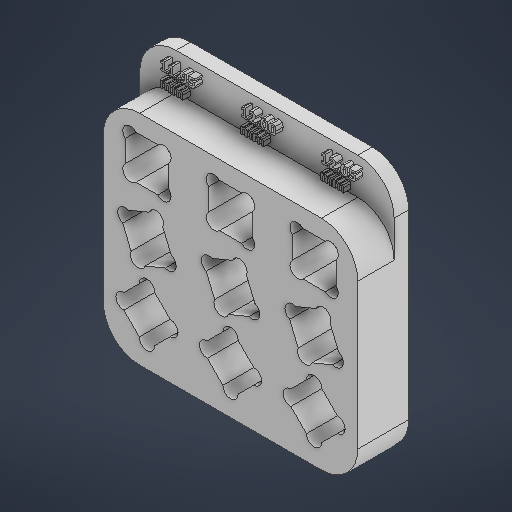
# Autodesk Inventor part: magnet_checker
Saved by Autodesk Inventor 2026.1 (Build 301233020, 233B)
## iProperties
Created: 2025-11-17
Part Number: magnet_checker
Material: Generic
Document SubType Name: Modeling
Designer: Carla Fernandez
Density: 1 g/cm^3
Appearance: Default
Author: Carla Fernandez
Autodesk Inventor part; units mm, degrees
ref_plane "YZ Plane" through (0, 0, 0) normal (1, 0, 0) x (0, 1, 0)
ref_plane "XZ Plane" through (0, 0, 0) normal (0, 1, 0) x (-1, 0, 0)
ref_plane "XY Plane" through (0, 0, 0) normal (0, 0, 1) x (1, 0, 0)
sketch "Sketch1" plane through (0, 0, 0) normal (0, 0, 1) x (1, 0, 0)
  line L0 (-35, 35) -> (35, 35)
  line L1 (35, 35) -> (35, -35)
  line L2 (35, -35) -> (-35, -35)
  line L3 (-35, -35) -> (-35, 35)
  point P0 (0, 0)
  point P1 (0, 35)
  point P2 (35, 0)
  dimension "d0" = 70
  dimension "d1" = 70
  constraints: 8 end point, 2 midpoint, 2 parallel, 1 horizontal, 1 horizontal alignment, 1 perpendicular, 1 vertical alignment
  measures "d0" distance of L2.end L0.start
  measures "d1" distance of L0.start L0.end
extrude "Extrusion1" add sketch "Sketch1" along normal blind 14
sketch "Sketch2" plane through (0, 0, 14) normal (0, 0, 1) x (1, 0, 0)
  line L0 (-28.975, 20) -> (-17.025, 20)
  line L1 (-17.025, 20) -> (-17.025, 8.05)
  line L2 (-17.025, 8.05) -> (-28.975, 8.05)
  line L3 (-28.975, 8.05) -> (-28.975, 20)
  line L4 (-35, 35) -> (-35, -35) projected
  line L5 (35, 35) -> (-35, 35) projected
  line L6 (-30.8067, -0.7414) -> (-19.7664, 3.8317)
  line L7 (-19.7664, 3.8317) -> (-15.1933, -7.2086)
  line L8 (-15.1933, -7.2086) -> (-26.2336, -11.7817)
  line L9 (-26.2336, -11.7817) -> (-30.8067, -0.7414)
  line L10 (-31.4499, -21.975) -> (-23, -13.5251)
  line L11 (-23, -13.5251) -> (-14.5501, -21.975)
  line L12 (-14.5501, -21.975) -> (-23, -30.4249)
  line L13 (-23, -30.4249) -> (-31.4499, -21.975)
  line L14 (-23, -30.4249) -> (-23, -13.5251) construction
  line L15 (-14.5501, -21.975) -> (-31.4499, -21.975) construction
  line L16 (-17.025, 20) -> (-28.975, 8.05) construction
  line L17 (-28.975, 20) -> (-17.025, 8.05) construction
  line L18 (-19.7664, 3.8317) -> (-26.2336, -11.7817) construction
  line L19 (-15.1933, -7.2086) -> (-30.8067, -0.7414) construction
  line L20 (-6, 20.025) -> (6, 20.025)
  line L21 (6, 20.025) -> (6, 8.025)
  line L22 (6, 8.025) -> (-6, 8.025)
  line L23 (-6, 8.025) -> (-6, 20.025)
  line L24 (-7.8394, -0.7278) -> (3.2472, 3.8644)
  line L25 (3.2472, 3.8644) -> (7.8394, -7.2222)
  line L26 (7.8394, -7.2222) -> (-3.2472, -11.8144)
  line L27 (-3.2472, -11.8144) -> (-7.8394, -0.7278)
  line L28 (-8.4853, -21.975) -> (0, -13.4897)
  line L29 (0, -13.4897) -> (8.4853, -21.975)
  line L30 (8.4853, -21.975) -> (0, -30.4603)
  line L31 (0, -30.4603) -> (-8.4853, -21.975)
  line L32 (0, -30.4603) -> (0, -13.4897) construction
  line L33 (8.4853, -21.975) -> (-8.4853, -21.975) construction
  line L34 (6, 20.025) -> (-6, 8.025) construction
  line L35 (-6, 20.025) -> (6, 8.025) construction
  line L36 (3.2472, 3.8644) -> (-3.2472, -11.8144) construction
  line L37 (7.8394, -7.2222) -> (-7.8394, -0.7278) construction
  line L38 (16.975, 20.05) -> (29.025, 20.05)
  line L39 (29.025, 20.05) -> (29.025, 8)
  line L40 (29.025, 8) -> (16.975, 8)
  line L41 (16.975, 8) -> (16.975, 20.05)
  line L42 (15.128, -0.7143) -> (26.2607, 3.897)
  line L43 (26.2607, 3.897) -> (30.872, -7.2357)
  line L44 (30.872, -7.2357) -> (19.7393, -11.847)
  line L45 (19.7393, -11.847) -> (15.128, -0.7143)
  line L46 (14.4794, -21.975) -> (23, -13.4544)
  line L47 (23, -13.4544) -> (31.5206, -21.975)
  line L48 (31.5206, -21.975) -> (23, -30.4956)
  line L49 (23, -30.4956) -> (14.4794, -21.975)
  line L50 (23, -30.4956) -> (23, -13.4544) construction
  line L51 (31.5206, -21.975) -> (14.4794, -21.975) construction
  line L52 (29.025, 20.05) -> (16.975, 8) construction
  line L53 (16.975, 20.05) -> (29.025, 8) construction
  line L54 (26.2607, 3.897) -> (19.7393, -11.847) construction
  line L55 (30.872, -7.2357) -> (15.128, -0.7143) construction
  line L56 (35, -35) -> (35, 35) construction
  point P0 (0, 0)
  point P1 (-23, 14.025)
  point P2 (-23, -21.975)
  point P3 (-23, 14.025)
  point P4 (-23, -3.975)
  point P5 (-23, -21.975)
  point P6 (0, 14.025)
  point P7 (0, -21.975)
  point P8 (0, 14.025)
  point P9 (0, -3.975)
  point P10 (0, -21.975)
  point P11 (23, 14.025)
  point P12 (23, -21.975)
  point P13 (23, 14.025)
  point P14 (23, -3.975)
  point P15 (23, -21.975)
  dimension "d4" = 11.95
  dimension "d6" = 15
  dimension "d9" = 18
  dimension "d10" = 18
  dimension "d11" = 22.5
  dimension "d12" = 12
  dimension "d15" = 18
  dimension "d16" = 18
  dimension "d17" = 22.5
  dimension "d18" = 12.05
  dimension "d21" = 18
  dimension "d22" = 18
  dimension "d23" = 22.5
  dimension "d24" = 12
  dimension "d25" = 12
  constraints: 108 end point, 18 midpoint, 18 parallel, 15 equal length, 15 perpendicular, 7 vertical alignment, 3 horizontal, 3 vertical, 2 horizontal alignment
  measures "d4" distance of L2.end L0.start
  measures "d6" distance between parallel lines of L0 L5
  measures "d9" distance of point (-23, -3.975) point (-23, 14.025)
  measures "d10" distance of point (-23, -21.975) point (-23, -3.975)
  measures "d11" angle of L2 L6
  measures "d12" distance of L23.start L20.start
  measures "d15" distance of point (0, -3.975) point (0, 14.025)
  measures "d16" distance of point (0, -21.975) point (0, -3.975)
  measures "d17" angle of L22 L24
  measures "d18" distance of L41.start L38.start
  measures "d21" distance of point (23, -3.975) point (23, 14.025)
  measures "d22" distance of point (23, -21.975) point (23, -3.975)
  measures "d23" angle of L40 L42
  measures "d24" distance from line of L56 point (23, 14.025)
  measures "d25" distance from line of L4 point (-23, 14.025)
extrude "Extrusion2" cut sketch "Sketch2" against normal blind 12
sketch "Sketch3" plane through (0, 0, 14) normal (0, 0, 1) x (1, 0, 0)
  circle A0 centre (-27.561, 18.586) radius 2.1
  circle A1 centre (-18.439, 18.586) radius 2.1
  circle A2 centre (-27.561, 9.464) radius 2.1
  circle A3 centre (-18.439, 9.464) radius 2.1
  line L0 (-28.975, 20) -> (-17.025, 8.05) construction
  line L1 (-28.975, 8.05) -> (-28.975, 20) construction
  line L2 (-28.975, 20) -> (-17.025, 20) construction
  line L3 (-17.025, 8.05) -> (-28.975, 8.05) construction
  line L4 (-17.025, 20) -> (-28.975, 8.05) construction
  line L5 (-30.8067, -0.7414) -> (-19.7664, 3.8317) construction
  line L6 (-15.1933, -7.2086) -> (-26.2336, -11.7817) construction
  line L7 (-19.7664, 3.8317) -> (-26.2336, -11.7817) construction
  line L8 (-26.2336, -11.7817) -> (-30.8067, -0.7414) construction
  line L9 (-15.1933, -7.2086) -> (-30.8067, -0.7414) construction
  line L10 (-31.4499, -21.975) -> (-23, -13.5251) construction
  line L11 (-23, -30.4249) -> (-31.4499, -21.975) construction
  line L12 (-23, -13.5251) -> (-23, -30.4249) construction
  line L13 (-14.5501, -21.975) -> (-23, -30.4249) construction
  line L14 (-31.4499, -21.975) -> (-14.5501, -21.975) construction
  circle A4 centre (-28.9592, -1.5066) radius 2.1
  circle A5 centre (-20.5316, 1.9842) radius 2.1
  circle A6 centre (-17.0408, -6.4434) radius 2.1
  circle A7 centre (-25.4684, -9.9342) radius 2.1
  line L15 (-19.7664, 3.8317) -> (-15.1933, -7.2086) projected
  circle A8 centre (-23, -15.5248) radius 2.1
  circle A9 centre (-16.5498, -21.975) radius 2.1
  circle A10 centre (-23, -28.4252) radius 2.1
  circle A11 centre (-29.4502, -21.975) radius 2.1
  line L16 (-23, -13.5251) -> (-14.5501, -21.975) projected
  circle A12 centre (-4.561, 18.586) radius 2.1
  circle A13 centre (-4.561, 9.464) radius 2.1
  circle A14 centre (4.561, 9.464) radius 2.1
  line L17 (-5.975, 20) -> (5.975, 8.05) construction
  line L18 (5.975, 20) -> (-5.975, 8.05) construction
  circle A15 centre (4.561, 18.586) radius 2.1
  line L19 (-8.4499, -21.975) -> (8.4499, -21.975) construction
  circle A16 centre (-6.4502, -21.975) radius 2.1
  circle A17 centre (6.4502, -21.975) radius 2.1
  circle A18 centre (0, -28.4252) radius 2.1
  line L20 (0, -13.5251) -> (0, -30.4249) construction
  circle A19 centre (2.4684, 1.9842) radius 2.1
  line L21 (7.8067, -7.2086) -> (-7.8067, -0.7414) construction
  circle A20 centre (5.9592, -6.4434) radius 2.1
  line L22 (3.2336, 3.8317) -> (-3.2336, -11.7817) construction
  circle A21 centre (-2.4684, -9.9342) radius 2.1
  circle A22 centre (0, -15.5248) radius 2.1
  circle A23 centre (-5.9592, -1.5066) radius 2.1
  circle A24 centre (18.439, 18.586) radius 2.1
  circle A25 centre (18.439, 9.464) radius 2.1
  circle A26 centre (27.561, 9.464) radius 2.1
  line L23 (17.025, 20) -> (28.975, 8.05) construction
  line L24 (28.975, 20) -> (17.025, 8.05) construction
  circle A27 centre (27.561, 18.586) radius 2.1
  line L25 (14.5501, -21.975) -> (31.4499, -21.975) construction
  circle A28 centre (16.5498, -21.975) radius 2.1
  circle A29 centre (29.4502, -21.975) radius 2.1
  circle A30 centre (23, -28.4252) radius 2.1
  line L26 (23, -13.5251) -> (23, -30.4249) construction
  circle A31 centre (25.4684, 1.9842) radius 2.1
  line L27 (30.8067, -7.2086) -> (15.1933, -0.7414) construction
  circle A32 centre (28.9592, -6.4434) radius 2.1
  line L28 (26.2336, 3.8317) -> (19.7664, -11.7817) construction
  circle A33 centre (20.5316, -9.9342) radius 2.1
  circle A34 centre (23, -15.5248) radius 2.1
  circle A35 centre (17.0408, -1.5066) radius 2.1
  point P0 (0, 0)
  dimension "d28" = 4.2
  dimension "d29" = 1.414
  dimension "d32" = 1.414
  dimension "d33" = 1.414
  dimension "d34" = 1.414
  dimension "d35" = 1.414
  dimension "d36" = 1.414
  dimension "d37" = 1.414
  dimension "d38" = 1.414
  dimension "d39" = 1.414
  dimension "d42" = 23
  constraints: 36 centre point, 36 end point, 33 point on line, 11 equal radius, 3 coincident, 2 horizontal, 2 horizontal alignment, 2 vertical alignment, 1 vertical, 86 other
  measures "d28" diameter of A0
  measures "d29" distance from line of A0.centre L1
  measures "d32" distance from line of L8 A4.centre
  measures "d33" distance from line of L15 A5.centre
  measures "d34" distance from line of L15 A6.centre
  measures "d35" distance from line of L6 A7.centre
  measures "d36" distance from line of L16 A8.centre
  measures "d37" distance from line of L13 A9.centre
  measures "d38" distance from line of A11.centre L10
  measures "d39" distance from line of L13 A10.centre
  measures "d42" distance of A0.centre A12.centre
extrude "Extrusion3" cut sketch "Sketch3" against normal blind 12
sketch "Sketch4" plane through (0, 0, 14) normal (0, 0, 1) x (1, 0, 0)
  circle A0 centre (-23, 14.025) radius 2
  line L0 (-28.975, 11.0166) -> (-28.975, 17.0334) projected
  line L1 (-26.0084, 20) -> (-19.9916, 20) projected
  circle A1 centre (-23, -3.975) radius 2
  circle A2 centre (-23, -21.975) radius 2
  circle A3 centre (0, 14.025) radius 2
  circle A4 centre (0, -3.975) radius 2
  circle A5 centre (0, -21.975) radius 2
  circle A6 centre (23, 14.025) radius 2
  circle A7 centre (23, -3.975) radius 2
  circle A8 centre (23, -21.975) radius 2
  point P0 (0, 0)
  point P1 (-28.975, 14.025)
  point P2 (-23, 20)
  dimension "d49" = 4
  dimension "d52" = 18
  dimension "d55" = 23
  constraints: 9 centre point, 2 midpoint, 1 horizontal, 1 horizontal alignment, 1 vertical, 1 vertical alignment, 16 other
  measures "d49" diameter of A0
  measures "d52" distance of A0.centre A1.centre
  measures "d55" distance of A0.centre A3.centre
extrude "Extrusion4" cut sketch "Sketch4" against normal through all
sketch "Sketch6" plane through (0, 0, 14) normal (0, 0, 1) x (1, 0, 0)
  line L0 (35, -35) -> (35, 35) projected
  line L1 (-35, 35) -> (35, 35)
  line L2 (35, 35) -> (35, 25)
  line L3 (35, 25) -> (-35, 25)
  line L4 (-35, 25) -> (-35, 35)
  point P0 (0, 0)
  dimension "d60" = 10
  constraints: 8 end point, 2 parallel, 1 horizontal, 1 perpendicular, 1 point on line
  measures "d60" distance between parallel lines of L3 L1
extrude "Extrusion5" cut sketch "Sketch6" against normal blind 10
sketch "Sketch5" plane through (0, 0, 4) normal (0, 0, 1) x (1, 0, 0)
  line L0 (-27.5814, 32.7858) -> (-13.7775, 32.7858) construction
  line L1 (-13.7775, 32.7858) -> (-13.7775, 28.2053) construction
  line L2 (-13.7775, 28.2053) -> (-27.5814, 28.2053) construction
  line L3 (-27.5814, 28.2053) -> (-27.5814, 32.7858) construction
  line L4 (-5.411, 32.7858) -> (5.411, 32.7858) construction
  line L5 (5.411, 32.7858) -> (5.411, 28.2053) construction
  line L6 (5.411, 28.2053) -> (-5.411, 28.2053) construction
  line L7 (-5.411, 28.2053) -> (-5.411, 32.7858) construction
  line L8 (16.6095, 32.7858) -> (30.4134, 32.7858) construction
  line L9 (30.4134, 32.7858) -> (30.4134, 28.2053) construction
  line L10 (30.4134, 28.2053) -> (16.6095, 28.2053) construction
  line L11 (16.6095, 28.2053) -> (16.6095, 32.7858) construction
  line L12 (-25.5704, 30.1943) -> (-27.248, 30.1943)
  line L13 (-27.248, 30.1943) -> (-27.248, 30.6369)
  line L14 (-27.248, 30.6369) -> (-26.7128, 30.6369)
  line L15 (-26.7128, 30.6369) -> (-26.7128, 31.981)
  line L16 (-26.7128, 31.981) -> (-27.248, 31.981)
  line L17 (-27.248, 31.981) -> (-27.248, 32.3947)
  spline S0 degree 2 poles (-27.248, 32.3947) (-27.1306, 32.3947) (-26.898, 32.4256) (-26.8281, 32.4585) knots 0 0 0 1 2 2 2
  spline S1 degree 2 poles (-26.8281, 32.4585) (-26.7478, 32.4997) (-26.6572, 32.6376) (-26.649, 32.7405) knots 0 0 0 1 2 2 2
  line L18 (-26.649, 32.7405) -> (-26.0932, 32.7405)
  line L19 (-26.0932, 32.7405) -> (-26.0932, 30.6369)
  line L20 (-26.0932, 30.6369) -> (-25.5704, 30.6369)
  line L21 (-25.5704, 30.6369) -> (-25.5704, 30.1943)
  line L22 (-23.3453, 30.1943) -> (-25.0229, 30.1943)
  line L23 (-25.0229, 30.1943) -> (-25.0229, 30.6369)
  line L24 (-25.0229, 30.6369) -> (-24.4877, 30.6369)
  line L25 (-24.4877, 30.6369) -> (-24.4877, 31.981)
  line L26 (-24.4877, 31.981) -> (-25.0229, 31.981)
  line L27 (-25.0229, 31.981) -> (-25.0229, 32.3947)
  spline S2 degree 2 poles (-25.0229, 32.3947) (-24.9056, 32.3947) (-24.673, 32.4256) (-24.603, 32.4585) knots 0 0 0 1 2 2 2
  spline S3 degree 2 poles (-24.603, 32.4585) (-24.5227, 32.4997) (-24.4321, 32.6376) (-24.4239, 32.7405) knots 0 0 0 1 2 2 2
  line L28 (-24.4239, 32.7405) -> (-23.8682, 32.7405)
  line L29 (-23.8682, 32.7405) -> (-23.8682, 30.6369)
  line L30 (-23.8682, 30.6369) -> (-23.3453, 30.6369)
  line L31 (-23.3453, 30.6369) -> (-23.3453, 30.1943)
  line L32 (-22.2853, 30.1943) -> (-22.8884, 30.1943)
  line L33 (-22.8884, 30.1943) -> (-22.8884, 30.8653)
  line L34 (-22.8884, 30.8653) -> (-22.2853, 30.8653)
  line L35 (-22.2853, 30.8653) -> (-22.2853, 30.1943)
  spline S4 degree 2 poles (-19.982, 31.6063) (-19.982, 31.2832) (-20.1323, 30.7439) (-20.2908, 30.5504) knots 0 0 0 1 2 2 2
  spline S5 degree 2 poles (-20.2908, 30.5504) (-20.4554, 30.3549) (-20.9412, 30.1449) (-21.2952, 30.1449) knots 0 0 0 1 2 2 2
  spline S6 degree 2 poles (-21.2952, 30.1449) (-21.4146, 30.1449) (-21.674, 30.1758) (-21.7172, 30.1881) knots 0 0 0 1 2 2 2
  line L36 (-21.7172, 30.1881) -> (-21.7172, 30.6863)
  line L37 (-21.7172, 30.6863) -> (-21.6678, 30.6863)
  spline S7 degree 2 poles (-21.6678, 30.6863) (-21.6204, 30.6616) (-21.4434, 30.608) (-21.2891, 30.608) knots 0 0 0 1 2 2 2
  spline S8 degree 2 poles (-21.2891, 30.608) (-21.1635, 30.608) (-20.9309, 30.6739) (-20.8486, 30.746) knots 0 0 0 1 2 2 2
  spline S9 degree 2 poles (-20.8486, 30.746) (-20.7601, 30.8221) (-20.6448, 31.0465) (-20.6242, 31.2153) knots 0 0 0 1 2 2 2
  spline S10 degree 2 poles (-20.6242, 31.2153) (-20.7601, 31.1309) (-20.9947, 31.0403) (-21.1697, 31.0403) knots 0 0 0 1 2 2 2
  spline S11 degree 2 poles (-21.1697, 31.0403) (-21.2993, 31.0403) (-21.5402, 31.1103) (-21.639, 31.1844) knots 0 0 0 1 2 2 2
  spline S12 degree 2 poles (-21.639, 31.1844) (-21.7707, 31.2852) (-21.9251, 31.6084) (-21.9251, 31.8636) knots 0 0 0 1 2 2 2
  spline S13 degree 2 poles (-21.9251, 31.8636) (-21.9251, 32.0633) (-21.7892, 32.3988) (-21.6657, 32.5223) knots 0 0 0 1 2 2 2
  spline S14 degree 2 poles (-21.6657, 32.5223) (-21.5422, 32.6458) (-21.1841, 32.7858) (-20.9638, 32.7858) knots 0 0 0 1 2 2 2
  spline S15 degree 2 poles (-20.9638, 32.7858) (-20.7415, 32.7858) (-20.3978, 32.6623) (-20.2743, 32.5326) knots 0 0 0 1 2 2 2
  spline S16 degree 2 poles (-20.2743, 32.5326) (-20.1302, 32.3885) (-19.982, 31.9316) (-19.982, 31.6063) knots 0 0 0 1 2 2 2
  spline S17 degree 2 poles (-20.6139, 31.701) (-20.6139, 31.9089) (-20.6839, 32.1765) (-20.7477, 32.2506) knots 0 0 0 1 2 2 2
  spline S18 degree 2 poles (-20.7477, 32.2506) (-20.7909, 32.3062) (-20.9021, 32.3535) (-20.9659, 32.3535) knots 0 0 0 1 2 2 2
  spline S19 degree 2 poles (-20.9659, 32.3535) (-21.0235, 32.3535) (-21.1306, 32.3082) (-21.18, 32.2506) knots 0 0 0 1 2 2 2
  spline S20 degree 2 poles (-21.18, 32.2506) (-21.2232, 32.2012) (-21.2849, 32.0098) (-21.2849, 31.8966) knots 0 0 0 1 2 2 2
  spline S21 degree 2 poles (-21.2849, 31.8966) (-21.2849, 31.7731) (-21.2211, 31.6146) (-21.1676, 31.5672) knots 0 0 0 1 2 2 2
  spline S22 degree 2 poles (-21.1676, 31.5672) (-21.112, 31.5199) (-20.9741, 31.4828) (-20.8877, 31.4828) knots 0 0 0 1 2 2 2
  spline S23 degree 2 poles (-20.8877, 31.4828) (-20.8156, 31.4828) (-20.6654, 31.522) (-20.618, 31.5425) knots 0 0 0 1 2 2 2
  spline S24 degree 2 poles (-20.618, 31.5425) (-20.618, 31.5611) (-20.6139, 31.631) (-20.6139, 31.701) knots 0 0 0 1 2 2 2
  spline S25 degree 2 poles (-17.7487, 31.0547) (-17.7487, 30.855) (-17.8845, 30.5175) (-18.0183, 30.396) knots 0 0 0 1 2 2 2
  spline S26 degree 2 poles (-18.0183, 30.396) (-18.1521, 30.2746) (-18.5185, 30.1408) (-18.7861, 30.1408) knots 0 0 0 1 2 2 2
  spline S27 degree 2 poles (-18.7861, 30.1408) (-19.0702, 30.1429) (-19.4777, 30.2355) (-19.6115, 30.2952) knots 0 0 0 1 2 2 2
  line L38 (-19.6115, 30.2952) -> (-19.6115, 30.8489)
  line L39 (-19.6115, 30.8489) -> (-19.5539, 30.8489)
  spline S28 degree 2 poles (-19.5539, 30.8489) (-19.5045, 30.8221) (-19.3851, 30.7521) (-19.2883, 30.7151) knots 0 0 0 1 2 2 2
  spline S29 degree 2 poles (-19.2883, 30.7151) (-19.1978, 30.6801) (-19.0105, 30.6327) (-18.8973, 30.6327) knots 0 0 0 1 2 2 2
  spline S30 degree 2 poles (-18.8973, 30.6327) (-18.7985, 30.6327) (-18.5679, 30.6821) (-18.4979, 30.748) knots 0 0 0 1 2 2 2
  spline S31 degree 2 poles (-18.4979, 30.748) (-18.4465, 30.7995) (-18.3888, 30.925) (-18.3888, 31.03) knots 0 0 0 1 2 2 2
  spline S32 degree 2 poles (-18.3888, 31.03) (-18.3888, 31.1206) (-18.4629, 31.2482) (-18.5226, 31.2873) knots 0 0 0 1 2 2 2
  spline S33 degree 2 poles (-18.5226, 31.2873) (-18.6091, 31.3449) (-18.8561, 31.3779) (-18.9446, 31.3779) knots 0 0 0 1 2 2 2
  spline S34 degree 2 poles (-18.9446, 31.3779) (-19.0846, 31.3779) (-19.3501, 31.3326) (-19.4468, 31.3079) knots 0 0 0 1 2 2 2
  line L40 (-19.4468, 31.3079) -> (-19.5024, 31.3079)
  line L41 (-19.5024, 31.3079) -> (-19.5024, 32.7343)
  line L42 (-19.5024, 32.7343) -> (-17.8187, 32.7343)
  line L43 (-17.8187, 32.7343) -> (-17.8187, 32.2547)
  line L44 (-17.8187, 32.2547) -> (-18.8993, 32.2547)
  line L45 (-18.8993, 32.2547) -> (-18.8993, 31.8328)
  spline S35 degree 2 poles (-18.8993, 31.8328) (-18.8479, 31.8369) (-18.7058, 31.841) (-18.6667, 31.841) knots 0 0 0 1 2 2 2
  spline S36 degree 2 poles (-18.6667, 31.841) (-18.4835, 31.841) (-18.1748, 31.7669) (-18.0533, 31.6907) knots 0 0 0 1 2 2 2
  spline S37 degree 2 poles (-18.0533, 31.6907) (-17.9092, 31.5961) (-17.7487, 31.2811) (-17.7487, 31.0547) knots 0 0 0 1 2 2 2
  line L46 (-25.0661, 26.0123) -> (-25.0661, 26.9694)
  spline S38 degree 2 poles (-25.0661, 26.9694) (-25.0661, 27.1114) (-25.0764, 27.3049) (-25.1011, 27.3667) knots 0 0 0 1 2 2 2
  spline S39 degree 2 poles (-25.1011, 27.3667) (-25.1279, 27.4284) (-25.2349, 27.484) (-25.3316, 27.484) knots 0 0 0 1 2 2 2
  spline S40 degree 2 poles (-25.3316, 27.484) (-25.3996, 27.484) (-25.5313, 27.4243) (-25.6095, 27.3687) knots 0 0 0 1 2 2 2
  line L47 (-25.6095, 27.3687) -> (-25.6095, 26.0123)
  line L48 (-25.6095, 26.0123) -> (-26.2106, 26.0123)
  line L49 (-26.2106, 26.0123) -> (-26.2106, 26.9694)
  spline S41 degree 2 poles (-26.2106, 26.9694) (-26.2106, 27.1094) (-26.2229, 27.3049) (-26.2476, 27.3667) knots 0 0 0 1 2 2 2
  spline S42 degree 2 poles (-26.2476, 27.3667) (-26.2744, 27.4284) (-26.3814, 27.484) (-26.4781, 27.484) knots 0 0 0 1 2 2 2
  spline S43 degree 2 poles (-26.4781, 27.484) (-26.5502, 27.484) (-26.6922, 27.4161) (-26.7581, 27.3687) knots 0 0 0 1 2 2 2
  line L50 (-26.7581, 27.3687) -> (-26.7581, 26.0123)
  line L51 (-26.7581, 26.0123) -> (-27.355, 26.0123)
  line L52 (-27.355, 26.0123) -> (-27.355, 27.9286)
  line L53 (-27.355, 27.9286) -> (-26.7581, 27.9286)
  line L54 (-26.7581, 27.9286) -> (-26.7581, 27.7166)
  spline S44 degree 2 poles (-26.7581, 27.7166) (-26.6119, 27.8401) (-26.3505, 27.9801) (-26.1879, 27.9801) knots 0 0 0 1 2 2 2
  spline S45 degree 2 poles (-26.1879, 27.9801) (-26.013, 27.9801) (-25.7454, 27.8133) (-25.6754, 27.6466) knots 0 0 0 1 2 2 2
  spline S46 degree 2 poles (-25.6754, 27.6466) (-25.5045, 27.8072) (-25.1999, 27.9801) (-25.0435, 27.9801) knots 0 0 0 1 2 2 2
  spline S47 degree 2 poles (-25.0435, 27.9801) (-24.9097, 27.9801) (-24.6977, 27.8957) (-24.6256, 27.8092) knots 0 0 0 1 2 2 2
  spline S48 degree 2 poles (-24.6256, 27.8092) (-24.5454, 27.7166) (-24.4651, 27.4634) (-24.4651, 27.2596) knots 0 0 0 1 2 2 2
  line L55 (-24.4651, 27.2596) -> (-24.4651, 26.0123)
  line L56 (-24.4651, 26.0123) -> (-25.0661, 26.0123)
  line L57 (-21.7357, 26.0123) -> (-21.7357, 26.9694)
  spline S49 degree 2 poles (-21.7357, 26.9694) (-21.7357, 27.1114) (-21.746, 27.3049) (-21.7707, 27.3667) knots 0 0 0 1 2 2 2
  spline S50 degree 2 poles (-21.7707, 27.3667) (-21.7975, 27.4284) (-21.9045, 27.484) (-22.0012, 27.484) knots 0 0 0 1 2 2 2
  spline S51 degree 2 poles (-22.0012, 27.484) (-22.0692, 27.484) (-22.2009, 27.4243) (-22.2791, 27.3687) knots 0 0 0 1 2 2 2
  line L58 (-22.2791, 27.3687) -> (-22.2791, 26.0123)
  line L59 (-22.2791, 26.0123) -> (-22.8802, 26.0123)
  line L60 (-22.8802, 26.0123) -> (-22.8802, 26.9694)
  spline S52 degree 2 poles (-22.8802, 26.9694) (-22.8802, 27.1094) (-22.8925, 27.3049) (-22.9172, 27.3667) knots 0 0 0 1 2 2 2
  spline S53 degree 2 poles (-22.9172, 27.3667) (-22.944, 27.4284) (-23.051, 27.484) (-23.1477, 27.484) knots 0 0 0 1 2 2 2
  spline S54 degree 2 poles (-23.1477, 27.484) (-23.2198, 27.484) (-23.3618, 27.4161) (-23.4277, 27.3687) knots 0 0 0 1 2 2 2
  line L61 (-23.4277, 27.3687) -> (-23.4277, 26.0123)
  line L62 (-23.4277, 26.0123) -> (-24.0246, 26.0123)
  line L63 (-24.0246, 26.0123) -> (-24.0246, 27.9286)
  line L64 (-24.0246, 27.9286) -> (-23.4277, 27.9286)
  line L65 (-23.4277, 27.9286) -> (-23.4277, 27.7166)
  spline S55 degree 2 poles (-23.4277, 27.7166) (-23.2815, 27.8401) (-23.0201, 27.9801) (-22.8575, 27.9801) knots 0 0 0 1 2 2 2
  spline S56 degree 2 poles (-22.8575, 27.9801) (-22.6826, 27.9801) (-22.415, 27.8133) (-22.345, 27.6466) knots 0 0 0 1 2 2 2
  spline S57 degree 2 poles (-22.345, 27.6466) (-22.1741, 27.8072) (-21.8695, 27.9801) (-21.7131, 27.9801) knots 0 0 0 1 2 2 2
  spline S58 degree 2 poles (-21.7131, 27.9801) (-21.5793, 27.9801) (-21.3673, 27.8957) (-21.2952, 27.8092) knots 0 0 0 1 2 2 2
  spline S59 degree 2 poles (-21.2952, 27.8092) (-21.215, 27.7166) (-21.1347, 27.4634) (-21.1347, 27.2596) knots 0 0 0 1 2 2 2
  line L66 (-21.1347, 27.2596) -> (-21.1347, 26.0123)
  line L67 (-21.1347, 26.0123) -> (-21.7357, 26.0123)
  line L68 (-3.4, 30.1943) -> (-5.0776, 30.1943)
  line L69 (-5.0776, 30.1943) -> (-5.0776, 30.6369)
  line L70 (-5.0776, 30.6369) -> (-4.5424, 30.6369)
  line L71 (-4.5424, 30.6369) -> (-4.5424, 31.981)
  line L72 (-4.5424, 31.981) -> (-5.0776, 31.981)
  line L73 (-5.0776, 31.981) -> (-5.0776, 32.3947)
  spline S60 degree 2 poles (-5.0776, 32.3947) (-4.9602, 32.3947) (-4.7276, 32.4256) (-4.6577, 32.4585) knots 0 0 0 1 2 2 2
  spline S61 degree 2 poles (-4.6577, 32.4585) (-4.5774, 32.4997) (-4.4868, 32.6376) (-4.4786, 32.7405) knots 0 0 0 1 2 2 2
  line L74 (-4.4786, 32.7405) -> (-3.9228, 32.7405)
  line L75 (-3.9228, 32.7405) -> (-3.9228, 30.6369)
  line L76 (-3.9228, 30.6369) -> (-3.4, 30.6369)
  line L77 (-3.4, 30.6369) -> (-3.4, 30.1943)
  line L78 (-1.0617, 30.1943) -> (-2.9287, 30.1943)
  line L79 (-2.9287, 30.1943) -> (-2.9287, 30.608)
  spline S62 degree 2 poles (-2.9287, 30.608) (-2.6919, 30.7974) (-2.3132, 31.1309) (-2.1712, 31.2811) knots 0 0 0 1 2 2 2
  spline S63 degree 2 poles (-2.1712, 31.2811) (-1.9839, 31.4767) (-1.8171, 31.7751) (-1.8171, 31.9316) knots 0 0 0 1 2 2 2
  spline S64 degree 2 poles (-1.8171, 31.9316) (-1.8171, 32.1086) (-2.0292, 32.298) (-2.2185, 32.298) knots 0 0 0 1 2 2 2
  spline S65 degree 2 poles (-2.2185, 32.298) (-2.3153, 32.298) (-2.4882, 32.2506) (-2.5767, 32.2136) knots 0 0 0 1 2 2 2
  spline S66 degree 2 poles (-2.5767, 32.2136) (-2.6631, 32.1745) (-2.7866, 32.0921) (-2.8175, 32.0715) knots 0 0 0 1 2 2 2
  line L80 (-2.8175, 32.0715) -> (-2.8669, 32.0715)
  line L81 (-2.8669, 32.0715) -> (-2.8669, 32.6252)
  spline S67 degree 2 poles (-2.8669, 32.6252) (-2.7599, 32.6767) (-2.3029, 32.7837) (-2.0909, 32.7837) knots 0 0 0 1 2 2 2
  spline S68 degree 2 poles (-2.0909, 32.7837) (-1.6381, 32.7837) (-1.1729, 32.3803) (-1.1729, 32.016) knots 0 0 0 1 2 2 2
  spline S69 degree 2 poles (-1.1729, 32.016) (-1.1729, 31.7916) (-1.3849, 31.3593) (-1.6298, 31.1123) knots 0 0 0 1 2 2 2
  spline S70 degree 2 poles (-1.6298, 31.1123) (-1.7842, 30.96) (-2.0744, 30.7233) (-2.1382, 30.6739) knots 0 0 0 1 2 2 2
  line L82 (-2.1382, 30.6739) -> (-1.0617, 30.6739)
  line L83 (-1.0617, 30.6739) -> (-1.0617, 30.1943)
  line L84 (-0.1149, 30.1943) -> (-0.718, 30.1943)
  line L85 (-0.718, 30.1943) -> (-0.718, 30.8653)
  line L86 (-0.718, 30.8653) -> (-0.1149, 30.8653)
  line L87 (-0.1149, 30.8653) -> (-0.1149, 30.1943)
  spline S71 degree 2 poles (2.2213, 31.4643) (2.2213, 31.135) (2.1164, 30.641) (1.999, 30.4743) knots 0 0 0 1 2 2 2
  spline S72 degree 2 poles (1.999, 30.4743) (1.8838, 30.3096) (1.5112, 30.1408) (1.2436, 30.1408) knots 0 0 0 1 2 2 2
  spline S73 degree 2 poles (1.2436, 30.1408) (0.974, 30.1408) (0.6035, 30.3096) (0.4861, 30.4784) knots 0 0 0 1 2 2 2
  spline S74 degree 2 poles (0.4861, 30.4784) (0.3688, 30.6451) (0.2638, 31.135) (0.2638, 31.4643) knots 0 0 0 1 2 2 2
  spline S75 degree 2 poles (0.2638, 31.4643) (0.2638, 31.8019) (0.3688, 32.2794) (0.4882, 32.4523) knots 0 0 0 1 2 2 2
  spline S76 degree 2 poles (0.4882, 32.4523) (0.6076, 32.6211) (0.9843, 32.7858) (1.2436, 32.7858) knots 0 0 0 1 2 2 2
  spline S77 degree 2 poles (1.2436, 32.7858) (1.5174, 32.7858) (1.8838, 32.6129) (2.0011, 32.442) knots 0 0 0 1 2 2 2
  spline S78 degree 2 poles (2.0011, 32.442) (2.1164, 32.2753) (2.2213, 31.7834) (2.2213, 31.4643) knots 0 0 0 1 2 2 2
  spline S79 degree 2 poles (1.5812, 31.4643) (1.5812, 31.9357) (1.4268, 32.3165) (1.2436, 32.3165) knots 0 0 0 1 2 2 2
  spline S80 degree 2 poles (1.2436, 32.3165) (1.0604, 32.3165) (0.904, 31.9357) (0.904, 31.4623) knots 0 0 0 1 2 2 2
  spline S81 degree 2 poles (0.904, 31.4623) (0.904, 30.9971) (1.0604, 30.6101) (1.2436, 30.6101) knots 0 0 0 1 2 2 2
  spline S82 degree 2 poles (1.2436, 30.6101) (1.4248, 30.6101) (1.5812, 30.9971) (1.5812, 31.4643) knots 0 0 0 1 2 2 2
  spline S83 degree 2 poles (4.4464, 31.4643) (4.4464, 31.135) (4.3414, 30.641) (4.2241, 30.4743) knots 0 0 0 1 2 2 2
  spline S84 degree 2 poles (4.2241, 30.4743) (4.1088, 30.3096) (3.7363, 30.1408) (3.4687, 30.1408) knots 0 0 0 1 2 2 2
  spline S85 degree 2 poles (3.4687, 30.1408) (3.199, 30.1408) (2.8285, 30.3096) (2.7112, 30.4784) knots 0 0 0 1 2 2 2
  spline S86 degree 2 poles (2.7112, 30.4784) (2.5939, 30.6451) (2.4889, 31.135) (2.4889, 31.4643) knots 0 0 0 1 2 2 2
  spline S87 degree 2 poles (2.4889, 31.4643) (2.4889, 31.8019) (2.5939, 32.2794) (2.7133, 32.4523) knots 0 0 0 1 2 2 2
  spline S88 degree 2 poles (2.7133, 32.4523) (2.8327, 32.6211) (3.2093, 32.7858) (3.4687, 32.7858) knots 0 0 0 1 2 2 2
  spline S89 degree 2 poles (3.4687, 32.7858) (3.7425, 32.7858) (4.1088, 32.6129) (4.2262, 32.442) knots 0 0 0 1 2 2 2
  spline S90 degree 2 poles (4.2262, 32.442) (4.3414, 32.2753) (4.4464, 31.7834) (4.4464, 31.4643) knots 0 0 0 1 2 2 2
  spline S91 degree 2 poles (3.8063, 31.4643) (3.8063, 31.9357) (3.6519, 32.3165) (3.4687, 32.3165) knots 0 0 0 1 2 2 2
  spline S92 degree 2 poles (3.4687, 32.3165) (3.2855, 32.3165) (3.1291, 31.9357) (3.1291, 31.4623) knots 0 0 0 1 2 2 2
  spline S93 degree 2 poles (3.1291, 31.4623) (3.1291, 30.9971) (3.2855, 30.6101) (3.4687, 30.6101) knots 0 0 0 1 2 2 2
  spline S94 degree 2 poles (3.4687, 30.6101) (3.6498, 30.6101) (3.8063, 30.9971) (3.8063, 31.4643) knots 0 0 0 1 2 2 2
  line L88 (-2.8957, 26.0123) -> (-2.8957, 26.9694)
  spline S95 degree 2 poles (-2.8957, 26.9694) (-2.8957, 27.1114) (-2.906, 27.3049) (-2.9307, 27.3667) knots 0 0 0 1 2 2 2
  spline S96 degree 2 poles (-2.9307, 27.3667) (-2.9575, 27.4284) (-3.0645, 27.484) (-3.1612, 27.484) knots 0 0 0 1 2 2 2
  spline S97 degree 2 poles (-3.1612, 27.484) (-3.2292, 27.484) (-3.3609, 27.4243) (-3.4391, 27.3687) knots 0 0 0 1 2 2 2
  line L89 (-3.4391, 27.3687) -> (-3.4391, 26.0123)
  line L90 (-3.4391, 26.0123) -> (-4.0402, 26.0123)
  line L91 (-4.0402, 26.0123) -> (-4.0402, 26.9694)
  spline S98 degree 2 poles (-4.0402, 26.9694) (-4.0402, 27.1094) (-4.0525, 27.3049) (-4.0772, 27.3667) knots 0 0 0 1 2 2 2
  spline S99 degree 2 poles (-4.0772, 27.3667) (-4.104, 27.4284) (-4.211, 27.484) (-4.3077, 27.484) knots 0 0 0 1 2 2 2
  spline S100 degree 2 poles (-4.3077, 27.484) (-4.3798, 27.484) (-4.5218, 27.4161) (-4.5877, 27.3687) knots 0 0 0 1 2 2 2
  line L92 (-4.5877, 27.3687) -> (-4.5877, 26.0123)
  line L93 (-4.5877, 26.0123) -> (-5.1846, 26.0123)
  line L94 (-5.1846, 26.0123) -> (-5.1846, 27.9286)
  line L95 (-5.1846, 27.9286) -> (-4.5877, 27.9286)
  line L96 (-4.5877, 27.9286) -> (-4.5877, 27.7166)
  spline S101 degree 2 poles (-4.5877, 27.7166) (-4.4415, 27.8401) (-4.1801, 27.9801) (-4.0175, 27.9801) knots 0 0 0 1 2 2 2
  spline S102 degree 2 poles (-4.0175, 27.9801) (-3.8426, 27.9801) (-3.575, 27.8133) (-3.505, 27.6466) knots 0 0 0 1 2 2 2
  spline S103 degree 2 poles (-3.505, 27.6466) (-3.3341, 27.8072) (-3.0295, 27.9801) (-2.8731, 27.9801) knots 0 0 0 1 2 2 2
  spline S104 degree 2 poles (-2.8731, 27.9801) (-2.7393, 27.9801) (-2.5273, 27.8957) (-2.4552, 27.8092) knots 0 0 0 1 2 2 2
  spline S105 degree 2 poles (-2.4552, 27.8092) (-2.375, 27.7166) (-2.2947, 27.4634) (-2.2947, 27.2596) knots 0 0 0 1 2 2 2
  line L97 (-2.2947, 27.2596) -> (-2.2947, 26.0123)
  line L98 (-2.2947, 26.0123) -> (-2.8957, 26.0123)
  line L99 (0.4347, 26.0123) -> (0.4347, 26.9694)
  spline S106 degree 2 poles (0.4347, 26.9694) (0.4347, 27.1114) (0.4244, 27.3049) (0.3997, 27.3667) knots 0 0 0 1 2 2 2
  spline S107 degree 2 poles (0.3997, 27.3667) (0.3729, 27.4284) (0.2659, 27.484) (0.1692, 27.484) knots 0 0 0 1 2 2 2
  spline S108 degree 2 poles (0.1692, 27.484) (0.1012, 27.484) (-0.0305, 27.4243) (-0.1087, 27.3687) knots 0 0 0 1 2 2 2
  line L100 (-0.1087, 27.3687) -> (-0.1087, 26.0123)
  line L101 (-0.1087, 26.0123) -> (-0.7098, 26.0123)
  line L102 (-0.7098, 26.0123) -> (-0.7098, 26.9694)
  spline S109 degree 2 poles (-0.7098, 26.9694) (-0.7098, 27.1094) (-0.7221, 27.3049) (-0.7468, 27.3667) knots 0 0 0 1 2 2 2
  spline S110 degree 2 poles (-0.7468, 27.3667) (-0.7736, 27.4284) (-0.8806, 27.484) (-0.9773, 27.484) knots 0 0 0 1 2 2 2
  spline S111 degree 2 poles (-0.9773, 27.484) (-1.0494, 27.484) (-1.1914, 27.4161) (-1.2573, 27.3687) knots 0 0 0 1 2 2 2
  line L103 (-1.2573, 27.3687) -> (-1.2573, 26.0123)
  line L104 (-1.2573, 26.0123) -> (-1.8542, 26.0123)
  line L105 (-1.8542, 26.0123) -> (-1.8542, 27.9286)
  line L106 (-1.8542, 27.9286) -> (-1.2573, 27.9286)
  line L107 (-1.2573, 27.9286) -> (-1.2573, 27.7166)
  spline S112 degree 2 poles (-1.2573, 27.7166) (-1.1111, 27.8401) (-0.8497, 27.9801) (-0.6871, 27.9801) knots 0 0 0 1 2 2 2
  spline S113 degree 2 poles (-0.6871, 27.9801) (-0.5122, 27.9801) (-0.2446, 27.8133) (-0.1746, 27.6466) knots 0 0 0 1 2 2 2
  spline S114 degree 2 poles (-0.1746, 27.6466) (-0.0037, 27.8072) (0.3009, 27.9801) (0.4573, 27.9801) knots 0 0 0 1 2 2 2
  spline S115 degree 2 poles (0.4573, 27.9801) (0.5911, 27.9801) (0.8031, 27.8957) (0.8752, 27.8092) knots 0 0 0 1 2 2 2
  spline S116 degree 2 poles (0.8752, 27.8092) (0.9554, 27.7166) (1.0357, 27.4634) (1.0357, 27.2596) knots 0 0 0 1 2 2 2
  line L108 (1.0357, 27.2596) -> (1.0357, 26.0123)
  line L109 (1.0357, 26.0123) -> (0.4347, 26.0123)
  line L110 (18.6205, 30.1943) -> (16.9429, 30.1943)
  line L111 (16.9429, 30.1943) -> (16.9429, 30.6369)
  line L112 (16.9429, 30.6369) -> (17.4781, 30.6369)
  line L113 (17.4781, 30.6369) -> (17.4781, 31.981)
  line L114 (17.4781, 31.981) -> (16.9429, 31.981)
  line L115 (16.9429, 31.981) -> (16.9429, 32.3947)
  spline S117 degree 2 poles (16.9429, 32.3947) (17.0603, 32.3947) (17.2929, 32.4256) (17.3628, 32.4585) knots 0 0 0 1 2 2 2
  spline S118 degree 2 poles (17.3628, 32.4585) (17.4431, 32.4997) (17.5337, 32.6376) (17.5419, 32.7405) knots 0 0 0 1 2 2 2
  line L116 (17.5419, 32.7405) -> (18.0977, 32.7405)
  line L117 (18.0977, 32.7405) -> (18.0977, 30.6369)
  line L118 (18.0977, 30.6369) -> (18.6205, 30.6369)
  line L119 (18.6205, 30.6369) -> (18.6205, 30.1943)
  line L120 (20.9588, 30.1943) -> (19.0919, 30.1943)
  line L121 (19.0919, 30.1943) -> (19.0919, 30.608)
  spline S119 degree 2 poles (19.0919, 30.608) (19.3286, 30.7974) (19.7073, 31.1309) (19.8493, 31.2811) knots 0 0 0 1 2 2 2
  spline S120 degree 2 poles (19.8493, 31.2811) (20.0366, 31.4767) (20.2034, 31.7751) (20.2034, 31.9316) knots 0 0 0 1 2 2 2
  spline S121 degree 2 poles (20.2034, 31.9316) (20.2034, 32.1086) (19.9914, 32.298) (19.802, 32.298) knots 0 0 0 1 2 2 2
  spline S122 degree 2 poles (19.802, 32.298) (19.7052, 32.298) (19.5323, 32.2506) (19.4438, 32.2136) knots 0 0 0 1 2 2 2
  spline S123 degree 2 poles (19.4438, 32.2136) (19.3574, 32.1745) (19.2339, 32.0921) (19.203, 32.0715) knots 0 0 0 1 2 2 2
  line L122 (19.203, 32.0715) -> (19.1536, 32.0715)
  line L123 (19.1536, 32.0715) -> (19.1536, 32.6252)
  spline S124 degree 2 poles (19.1536, 32.6252) (19.2606, 32.6767) (19.7176, 32.7837) (19.9296, 32.7837) knots 0 0 0 1 2 2 2
  spline S125 degree 2 poles (19.9296, 32.7837) (20.3824, 32.7837) (20.8476, 32.3803) (20.8476, 32.016) knots 0 0 0 1 2 2 2
  spline S126 degree 2 poles (20.8476, 32.016) (20.8476, 31.7916) (20.6356, 31.3593) (20.3907, 31.1123) knots 0 0 0 1 2 2 2
  spline S127 degree 2 poles (20.3907, 31.1123) (20.2363, 30.96) (19.9461, 30.7233) (19.8823, 30.6739) knots 0 0 0 1 2 2 2
  line L124 (19.8823, 30.6739) -> (20.9588, 30.6739)
  line L125 (20.9588, 30.6739) -> (20.9588, 30.1943)
  line L126 (21.9056, 30.1943) -> (21.3025, 30.1943)
  line L127 (21.3025, 30.1943) -> (21.3025, 30.8653)
  line L128 (21.3025, 30.8653) -> (21.9056, 30.8653)
  line L129 (21.9056, 30.8653) -> (21.9056, 30.1943)
  spline S128 degree 2 poles (24.2418, 31.4643) (24.2418, 31.135) (24.1369, 30.641) (24.0195, 30.4743) knots 0 0 0 1 2 2 2
  spline S129 degree 2 poles (24.0195, 30.4743) (23.9043, 30.3096) (23.5317, 30.1408) (23.2641, 30.1408) knots 0 0 0 1 2 2 2
  spline S130 degree 2 poles (23.2641, 30.1408) (22.9945, 30.1408) (22.624, 30.3096) (22.5067, 30.4784) knots 0 0 0 1 2 2 2
  spline S131 degree 2 poles (22.5067, 30.4784) (22.3893, 30.6451) (22.2844, 31.135) (22.2844, 31.4643) knots 0 0 0 1 2 2 2
  spline S132 degree 2 poles (22.2844, 31.4643) (22.2844, 31.8019) (22.3893, 32.2794) (22.5087, 32.4523) knots 0 0 0 1 2 2 2
  spline S133 degree 2 poles (22.5087, 32.4523) (22.6281, 32.6211) (23.0048, 32.7858) (23.2641, 32.7858) knots 0 0 0 1 2 2 2
  spline S134 degree 2 poles (23.2641, 32.7858) (23.5379, 32.7858) (23.9043, 32.6129) (24.0216, 32.442) knots 0 0 0 1 2 2 2
  spline S135 degree 2 poles (24.0216, 32.442) (24.1369, 32.2753) (24.2418, 31.7834) (24.2418, 31.4643) knots 0 0 0 1 2 2 2
  spline S136 degree 2 poles (23.6017, 31.4643) (23.6017, 31.9357) (23.4473, 32.3165) (23.2641, 32.3165) knots 0 0 0 1 2 2 2
  spline S137 degree 2 poles (23.2641, 32.3165) (23.0809, 32.3165) (22.9245, 31.9357) (22.9245, 31.4623) knots 0 0 0 1 2 2 2
  spline S138 degree 2 poles (22.9245, 31.4623) (22.9245, 30.9971) (23.0809, 30.6101) (23.2641, 30.6101) knots 0 0 0 1 2 2 2
  spline S139 degree 2 poles (23.2641, 30.6101) (23.4453, 30.6101) (23.6017, 30.9971) (23.6017, 31.4643) knots 0 0 0 1 2 2 2
  spline S140 degree 2 poles (26.4422, 31.0547) (26.4422, 30.855) (26.3064, 30.5175) (26.1726, 30.396) knots 0 0 0 1 2 2 2
  spline S141 degree 2 poles (26.1726, 30.396) (26.0388, 30.2746) (25.6724, 30.1408) (25.4048, 30.1408) knots 0 0 0 1 2 2 2
  spline S142 degree 2 poles (25.4048, 30.1408) (25.1208, 30.1429) (24.7132, 30.2355) (24.5794, 30.2952) knots 0 0 0 1 2 2 2
  line L130 (24.5794, 30.2952) -> (24.5794, 30.8489)
  line L131 (24.5794, 30.8489) -> (24.637, 30.8489)
  spline S143 degree 2 poles (24.637, 30.8489) (24.6864, 30.8221) (24.8058, 30.7521) (24.9026, 30.7151) knots 0 0 0 1 2 2 2
  spline S144 degree 2 poles (24.9026, 30.7151) (24.9931, 30.6801) (25.1804, 30.6327) (25.2937, 30.6327) knots 0 0 0 1 2 2 2
  spline S145 degree 2 poles (25.2937, 30.6327) (25.3925, 30.6327) (25.623, 30.6821) (25.693, 30.748) knots 0 0 0 1 2 2 2
  spline S146 degree 2 poles (25.693, 30.748) (25.7444, 30.7995) (25.8021, 30.925) (25.8021, 31.03) knots 0 0 0 1 2 2 2
  spline S147 degree 2 poles (25.8021, 31.03) (25.8021, 31.1206) (25.728, 31.2482) (25.6683, 31.2873) knots 0 0 0 1 2 2 2
  spline S148 degree 2 poles (25.6683, 31.2873) (25.5818, 31.3449) (25.3348, 31.3779) (25.2463, 31.3779) knots 0 0 0 1 2 2 2
  spline S149 degree 2 poles (25.2463, 31.3779) (25.1063, 31.3779) (24.8408, 31.3326) (24.7441, 31.3079) knots 0 0 0 1 2 2 2
  line L132 (24.7441, 31.3079) -> (24.6885, 31.3079)
  line L133 (24.6885, 31.3079) -> (24.6885, 32.7343)
  line L134 (24.6885, 32.7343) -> (26.3722, 32.7343)
  line L135 (26.3722, 32.7343) -> (26.3722, 32.2547)
  line L136 (26.3722, 32.2547) -> (25.2916, 32.2547)
  line L137 (25.2916, 32.2547) -> (25.2916, 31.8328)
  spline S150 degree 2 poles (25.2916, 31.8328) (25.3431, 31.8369) (25.4851, 31.841) (25.5242, 31.841) knots 0 0 0 1 2 2 2
  spline S151 degree 2 poles (25.5242, 31.841) (25.7074, 31.841) (26.0161, 31.7669) (26.1376, 31.6907) knots 0 0 0 1 2 2 2
  spline S152 degree 2 poles (26.1376, 31.6907) (26.2817, 31.5961) (26.4422, 31.2811) (26.4422, 31.0547) knots 0 0 0 1 2 2 2
  line L138 (19.1248, 26.0123) -> (19.1248, 26.9694)
  spline S153 degree 2 poles (19.1248, 26.9694) (19.1248, 27.1114) (19.1145, 27.3049) (19.0898, 27.3667) knots 0 0 0 1 2 2 2
  spline S154 degree 2 poles (19.0898, 27.3667) (19.063, 27.4284) (18.956, 27.484) (18.8593, 27.484) knots 0 0 0 1 2 2 2
  spline S155 degree 2 poles (18.8593, 27.484) (18.7913, 27.484) (18.6596, 27.4243) (18.5814, 27.3687) knots 0 0 0 1 2 2 2
  line L139 (18.5814, 27.3687) -> (18.5814, 26.0123)
  line L140 (18.5814, 26.0123) -> (17.9803, 26.0123)
  line L141 (17.9803, 26.0123) -> (17.9803, 26.9694)
  spline S156 degree 2 poles (17.9803, 26.9694) (17.9803, 27.1094) (17.968, 27.3049) (17.9433, 27.3667) knots 0 0 0 1 2 2 2
  spline S157 degree 2 poles (17.9433, 27.3667) (17.9165, 27.4284) (17.8095, 27.484) (17.7128, 27.484) knots 0 0 0 1 2 2 2
  spline S158 degree 2 poles (17.7128, 27.484) (17.6407, 27.484) (17.4987, 27.4161) (17.4328, 27.3687) knots 0 0 0 1 2 2 2
  line L142 (17.4328, 27.3687) -> (17.4328, 26.0123)
  line L143 (17.4328, 26.0123) -> (16.8359, 26.0123)
  line L144 (16.8359, 26.0123) -> (16.8359, 27.9286)
  line L145 (16.8359, 27.9286) -> (17.4328, 27.9286)
  line L146 (17.4328, 27.9286) -> (17.4328, 27.7166)
  spline S159 degree 2 poles (17.4328, 27.7166) (17.579, 27.8401) (17.8404, 27.9801) (18.003, 27.9801) knots 0 0 0 1 2 2 2
  spline S160 degree 2 poles (18.003, 27.9801) (18.1779, 27.9801) (18.4455, 27.8133) (18.5155, 27.6466) knots 0 0 0 1 2 2 2
  spline S161 degree 2 poles (18.5155, 27.6466) (18.6864, 27.8072) (18.991, 27.9801) (19.1474, 27.9801) knots 0 0 0 1 2 2 2
  spline S162 degree 2 poles (19.1474, 27.9801) (19.2812, 27.9801) (19.4932, 27.8957) (19.5653, 27.8092) knots 0 0 0 1 2 2 2
  spline S163 degree 2 poles (19.5653, 27.8092) (19.6455, 27.7166) (19.7258, 27.4634) (19.7258, 27.2596) knots 0 0 0 1 2 2 2
  line L147 (19.7258, 27.2596) -> (19.7258, 26.0123)
  line L148 (19.7258, 26.0123) -> (19.1248, 26.0123)
  line L149 (22.4552, 26.0123) -> (22.4552, 26.9694)
  spline S164 degree 2 poles (22.4552, 26.9694) (22.4552, 27.1114) (22.4449, 27.3049) (22.4202, 27.3667) knots 0 0 0 1 2 2 2
  spline S165 degree 2 poles (22.4202, 27.3667) (22.3934, 27.4284) (22.2864, 27.484) (22.1897, 27.484) knots 0 0 0 1 2 2 2
  spline S166 degree 2 poles (22.1897, 27.484) (22.1217, 27.484) (21.99, 27.4243) (21.9118, 27.3687) knots 0 0 0 1 2 2 2
  line L150 (21.9118, 27.3687) -> (21.9118, 26.0123)
  line L151 (21.9118, 26.0123) -> (21.3108, 26.0123)
  line L152 (21.3108, 26.0123) -> (21.3108, 26.9694)
  spline S167 degree 2 poles (21.3108, 26.9694) (21.3108, 27.1094) (21.2984, 27.3049) (21.2737, 27.3667) knots 0 0 0 1 2 2 2
  spline S168 degree 2 poles (21.2737, 27.3667) (21.2469, 27.4284) (21.1399, 27.484) (21.0432, 27.484) knots 0 0 0 1 2 2 2
  spline S169 degree 2 poles (21.0432, 27.484) (20.9711, 27.484) (20.8291, 27.4161) (20.7632, 27.3687) knots 0 0 0 1 2 2 2
  line L153 (20.7632, 27.3687) -> (20.7632, 26.0123)
  line L154 (20.7632, 26.0123) -> (20.1663, 26.0123)
  line L155 (20.1663, 26.0123) -> (20.1663, 27.9286)
  line L156 (20.1663, 27.9286) -> (20.7632, 27.9286)
  line L157 (20.7632, 27.9286) -> (20.7632, 27.7166)
  spline S170 degree 2 poles (20.7632, 27.7166) (20.9094, 27.8401) (21.1708, 27.9801) (21.3334, 27.9801) knots 0 0 0 1 2 2 2
  spline S171 degree 2 poles (21.3334, 27.9801) (21.5084, 27.9801) (21.7759, 27.8133) (21.8459, 27.6466) knots 0 0 0 1 2 2 2
  spline S172 degree 2 poles (21.8459, 27.6466) (22.0168, 27.8072) (22.3214, 27.9801) (22.4778, 27.9801) knots 0 0 0 1 2 2 2
  spline S173 degree 2 poles (22.4778, 27.9801) (22.6116, 27.9801) (22.8236, 27.8957) (22.8957, 27.8092) knots 0 0 0 1 2 2 2
  spline S174 degree 2 poles (22.8957, 27.8092) (22.976, 27.7166) (23.0562, 27.4634) (23.0562, 27.2596) knots 0 0 0 1 2 2 2
  line L158 (23.0562, 27.2596) -> (23.0562, 26.0123)
  line L159 (23.0562, 26.0123) -> (22.4552, 26.0123)
  point P0 (0, 0)
  point P1 (0, 32.7858)
  dimension "d0" = 70
  dimension "d1" = 70
  constraints: 2 horizontal alignment, 1 midpoint, 1 vertical alignment, 6 other
emboss "Emboss1" sketch "Sketch5" operation add depth 2 direction (0, 0, -1)
fillet "Fillet1" radius 10 6 edges at (35, 25, 9) (35, 35, 2) (-35, 35, 2) (-35, 25, 9) (-35, -35, 7) (35, -35, 7)
body "Solid1"
